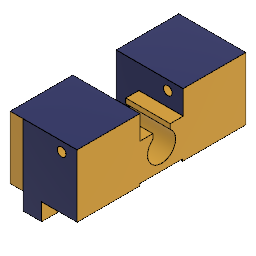
Lock_milling_jig_core_v1 v1 (Autodesk Fusion 360 design; units mm, degrees)
Autodesk Fusion 360 part; units mm, degrees
sketch "Sketch1" plane through (0, 0, 0) normal (0, 1, 0) x (1, 0, 0)
  line L0 (25, -14.9524) -> (-25, -14.9524)
  line L1 (-25, -14.9524) -> (-25, 0)
  line L2 (-25, 0) -> (25, 0)
  line L3 (25, 0) -> (25, -14.9524)
  constraint horizontal L0
  constraint vertical L1
  constraint horizontal L2
  constraint vertical L3
surface "Extrude1" add extruded along (0, 1, 0) between 0 and 50 path "Sketch1" along L2 L3 L0 L1 makes body 1
delete_face "SurfaceDeleteFace1" leaving the opening 1 faces at (8.3333, 16.6667, 14.9524) on bodies 1
delete_face "SurfaceDeleteFace2" leaving the opening 1 faces at (25, 16.6667, 4.9841) on bodies 1
delete_face "SurfaceDeleteFace3" leaving the opening 1 faces at (-8.3333, 16.6667, 0) on bodies 1
delete_face "SurfaceDeleteFace4" leaving the opening 1 faces at (-25, 16.6667, 9.9683) on bodies 1
sketch "Sketch2" plane through (0, 0, 0) normal (0, 1, 0) x (1, 0, 0)
  line L0 (-10, -10) -> (10, -10)
  line L1 (10, -10) -> (10, 0)
  line L2 (10, 0) -> (-10, 0)
  line L3 (-10, 0) -> (-10, -10)
  constraint horizontal L0
  constraint vertical L1
  constraint horizontal L2
  constraint vertical L3
extrude "Extrude2" add sketch "Sketch2" along normal mid plane 50 separate body makes body 2
hole "Hole1" at (-10, 0.0115, 9.2232) direction (1, 0, 0) diameter 12.9 depth 22 tip angle 180 bodies 2
hole "Hole2" at (0, 15.7073, 10) direction (0, 0, -1) diameter 4 depth 12 tip angle 118 counterbore diameter 6 counterbore depth 1 bodies 2
hole "Hole3" at (0, -15.6958, 10) direction (0, 0, -1) diameter 4 depth 12 tip angle 118 counterbore diameter 6 counterbore depth 1 bodies 2
sketch "Sketch3" plane through (0, 0, 0) normal (1, 0, 0) x (0, 1, 0)
  line L0 (6, 10, -10) -> (-6, 10, -10)
  line L1 (-6, 10, -10) -> (-6, 2, -10)
  line L2 (-6, 2, -10) -> (6, 2, -10)
  line L3 (6, 2, -10) -> (6, 10, -10)
extrude "Extrude3" cut sketch "Sketch3" along normal blind 10 contours L0 L1 L2 L3 in plane through (-10, 0, 0) normal (1, 0, 0) bodies 2
sketch "Sketch4" plane through (0, 0, 0) normal (0, 0, -1) x (1, 0, 0)
  circle A0 centre (0, 15.6958) radius 2
  circle A1 centre (0, -15.7073) radius 2
  line L0 (-10, 25) -> (-10, -25)
  line L1 (-10, -25) -> (10, -25)
  line L2 (10, -25) -> (10, 25)
  line L3 (10, 25) -> (-10, 25)
extrude "Extrude4" add 1 faces at (7.6639, 15.782, 10) along direction (0, 0, 1) blind 2 on bodies 2 bodies 2
extrude "Extrude5" add 1 faces at (7.6639, -15.6211, 10) along direction (0, 0, 1) blind 2 on bodies 2 bodies 2
extrude "Extrude6" cut 1 faces at (-6.6667, -2, 2) along direction (0, 0, -1) blind 1 on bodies 2 bodies 2
extrude "Extrude7" add sketch "Sketch4" along normal blind 2 bodies 2
chamfer "Chamfer1" distance 0.4 angle 45 1 edges at (-2.797, -14.6109, 12) on bodies 2
chamfer "Chamfer2" distance 0.4 angle 45 1 edges at (-2.797, 16.7921, 12) on bodies 2
chamfer "Chamfer3" distance 0.5 angle 45 1 edges at (-10, -25, 5) on bodies 2
chamfer "Chamfer4" distance 0.5 angle 45 1 edges at (10, -25, 5) on bodies 2
chamfer "Chamfer5" distance 0.5 angle 45 1 edges at (10, 25, 5) on bodies 2
chamfer "Chamfer6" distance 0.5 angle 45 1 edges at (-10, 25, 5) on bodies 2
sketch "Sketch5" plane through (0, 0, 0) normal (1, 0, 0) x (0, 1, 0)
  line L0 (10, 15) -> (-10, 15)
  line L1 (-10, 15) -> (-10, 1)
  line L2 (-10, 1) -> (10, 1)
  line L3 (10, 1) -> (10, 15)
  constraint horizontal L0
  constraint vertical L1
  constraint horizontal L2
  constraint vertical L3
extrude "Extrude8" cut sketch "Sketch5" against normal blind 12 bodies 2
extrude "Extrude9" add 1 faces at (7.2673, -4.9427, -2) along direction (0, 0, -1) blind 2 on bodies 2 bodies 2
chamfer "Chamfer7" distance 0.5 angle 45 1 edges at (-10, 10, 6.5) on bodies 2
chamfer "Chamfer8" distance 0.5 angle 45 1 edges at (-10, 0.25, 1) on bodies 2
chamfer "Chamfer9" distance 0.5 angle 45 1 edges at (-10, -10, 6.25) on bodies 2
extrude "Extrude10" add 1 faces at (3.3333, 6.4145, 10.6667) along direction (0, -1, 0) blind 2 on bodies 2 bodies 2
extrude "Extrude11" add 1 faces at (3.3333, -6.3916, 10.6667) along direction (0, 1, 0) blind 2 on bodies 2 bodies 2
extrude "Extrude12" add 1 faces at (7.7968, 14.7892, 12) along direction (0, 0, 1) blind 3 on bodies 2 bodies 2
extrude "Extrude13" add 1 faces at (7.7968, -14.7778, 12) along direction (0, 0, 1) blind 3 on bodies 2 bodies 2
sketch "Sketch6" plane through (10, 0, 0) normal (1, 0, 0) x (0, 1, 0)
  line L0 (24.5, -4) -> (24.5, 15)
  line L1 (24.5, 15) -> (4.4145, 15)
  line L2 (4.4145, 15) -> (4.4145, 10)
  line L3 (4.4145, 10) -> (6.4145, 10)
  arc A0 (-6.3916, 10) -> (6.4145, 10) centre (0.0115, 9.2232) ccw
  line L4 (-6.3916, 10) -> (-4.3916, 10)
  line L5 (-4.3916, 10) -> (-4.3916, 15)
  line L6 (-4.3916, 15) -> (-24.5, 15)
  line L7 (-24.5, 15) -> (-24.5, -4)
  line L8 (-24.5, -4) -> (24.5, -4)
  circle A1 centre (0.0115, 9.2232) radius 6.4
  constraint concentric A0 A1
extrude "Extrude14" cut sketch "Sketch6" against normal blind 19 contours L2 L3 A1 | L4 L5 A1 bodies 2
extrude "Extrude15" add 1 faces at (7.7968, 14.7892, 15) along direction (0, 0, 1) blind 4 on bodies 2 bodies 2
extrude "Extrude16" add 1 faces at (7.7968, -14.7778, 15) along direction (0, 0, 1) blind 4 on bodies 2 bodies 2
delete_face "DeleteFace1" 1 faces at (-9.6667, 10.1667, 10.6667) on bodies 2
delete_face "DeleteFace2" 1 faces at (-9.8333, -3.5, 0.6667) on bodies 2
delete_face "DeleteFace3" 1 faces at (-9.6667, -10.1667, 13) on bodies 2
delete_face "DeleteFace4" 1 faces at (-9.8333, 24.6667, 11.3333) on bodies 2
delete_face "DeleteFace5" 1 faces at (-9.8333, -24.6667, 3.6667) on bodies 2
extrude "Extrude17" add 1 faces at (-10, 20, 5.3333) along direction (-1, 0, 0) blind 8 on bodies 2 bodies 2
extrude "Extrude18" add 1 faces at (-13.1302, 16.9871, 19) along direction (0, 0, 1) blind 3 on bodies 2 bodies 2
extrude "Extrude19" add 1 faces at (-13.1302, -16.9833, 19) along direction (0, 0, 1) blind 3 on bodies 2 bodies 2
sketch "Sketch7" plane through (10, 0, 0) normal (1, 0, 0) x (0, 1, 0)
  arc A0 (6.3642, 10) -> (4.4145, 13.8679) centre (0.0115, 9.2232) ccw
  line L0 (-4.3916, 13.8679) -> (-4.3916, 22)
  line L1 (-4.3916, 22) -> (-24.5, 22)
  line L2 (-24.5, 22) -> (-24.5, -4)
  line L3 (-24.5, -4) -> (24.5, -4)
  line L4 (24.5, -4) -> (24.5, 22)
  line L5 (24.5, 22) -> (4.4145, 22)
  line L6 (4.4145, 22) -> (4.4145, 13.8679)
  line L7 (-8, 23) -> (8, 23)
  line L8 (8, 23) -> (8, 16)
  line L9 (8, 16) -> (-8, 16)
  line L10 (-8, 16) -> (-8, 23)
  line L11 (6.3642, 10) -> (6.4145, 10)
  arc A1 (-6.3916, 10) -> (6.4145, 10) centre (0.0115, 9.2232) ccw
  line L12 (-6.3916, 10) -> (-6.3412, 10)
  arc A2 (-4.3916, 13.8679) -> (-6.3412, 10) centre (0.0115, 9.2232) ccw
  constraint horizontal L7
  constraint vertical L8
  constraint horizontal L9
  constraint vertical L10
extrude "Extrude20" cut sketch "Sketch7" against normal blind 13 contours L5 L6 L8 L9 | L0 L1 L9 L10 bodies 2
hole "Hole4" at (-7.848, -25, 14.6725) direction (0, 1, 0) diameter 4 depth 50 tip angle 180 bodies 2
extrude "Extrude21" cut 1 faces at (-12.5508, -4.8564, -4) along direction (0, 0, 1) blind 2 on bodies 2 bodies 2
extrude "Extrude22" cut 1 faces at (-18, 20, 7) along direction (1, 0, 0) blind 3 on bodies 2 bodies 2
extrude "Extrude23" cut 1 faces at (6.6667, 8, 20) along direction (0, 1, 0) blind 2 on bodies 2 bodies 2
extrude "Extrude24" cut 1 faces at (6.6667, -8, 18) along direction (0, -1, 0) blind 2 on bodies 2 bodies 2
delete_face "DeleteFace6" 1 faces at (-7.6488, 15, 12.6824) on bodies 2
delete_face "DeleteFace7" 2 faces at (0, 13.7073, -1.3333) (2, 15.7073, 6) on bodies 2
delete_face "DeleteFace8" 2 faces at (0, -17.6958, -1.3333) (2, -15.6958, 6) on bodies 2
delete_face "DeleteFace9" 1 faces at (0.1695, -19.0916, 18.6667) on bodies 2
delete_face "DeleteFace10" 1 faces at (0.1695, 12.3115, 18.6667) on bodies 2
delete_face "DeleteFace11" 1 faces at (-7.6488, -20, 12.6824) on bodies 2
extrude "Extrude25" add 1 faces at (1.5, 15, 22) along direction (0, 0, 1) blind 4 on bodies 2 bodies 2
extrude "Extrude26" add 1 faces at (1.5, -15, 22) along direction (0, 0, 1) blind 5 on bodies 2 bodies 2
hole "Hole5" at (-9.451, -25, 21.8297) direction (0, 1, 0) diameter 4 depth 55 tip angle 118 bodies 2
extrude "Extrude27" add 1 faces at (0, -8.8121, 8.6844) along direction (-1, 0, 0) blind 9 on bodies 2 bodies 2
delete_face "DeleteFace12" 1 faces at (-10.9194, -20, 20.4719) on bodies 2
delete_face "DeleteFace13" 1 faces at (-10.9194, 20, 20.4719) on bodies 2
delete_face "DeleteFace14" 1 faces at (9.6667, -24.8333, 7.6667) on bodies 2
delete_face "DeleteFace15" 1 faces at (9.8333, 24.6667, 7.3333) on bodies 2
sketch "Sketch8" plane through (-15, 0, 0) normal (-1, 0, 0) x (0, -1, 0)
  line L0 (-25, -2) -> (25, -2)
  line L1 (25, -2) -> (25, 27)
  line L2 (25, 27) -> (10, 27)
  line L3 (10, 27) -> (10, 1)
  line L4 (10, 1) -> (-10, 1)
  line L5 (-10, 1) -> (-10, 26)
  line L6 (-10, 26) -> (-25, 26)
  line L7 (-25, 26) -> (-25, -2)
  line L8 (-25, -2) -> (25, -2)
  line L9 (25, -2) -> (25, -10)
  line L10 (25, -10) -> (-25, -10)
  line L11 (-25, -10) -> (-25, -2)
  constraint horizontal L8
  constraint vertical L9
  constraint horizontal L10
  constraint vertical L11
  constraint coincident L0.start L7.end
extrude "Extrude28" add sketch "Sketch8" against normal blind 9 contours L0 L8 L9 L10 L11 bodies 2
sketch "Sketch9" plane through (-15, 0, 0) normal (-1, 0, 0) x (0, -1, 0)
  line L0 (25, -10) -> (25, 27)
  line L1 (25, 27) -> (10, 27)
  line L2 (10, 27) -> (10, 1)
  line L3 (10, 1) -> (-10, 1)
  line L4 (-10, 1) -> (-10, 26)
  line L5 (-10, 26) -> (-25, 26)
  line L6 (-25, 26) -> (-25, -10)
  line L7 (-25, -10) -> (25, -10)
  line L8 (-10, -3) -> (10, -3)
  line L9 (10, -3) -> (10, -10)
  line L10 (10, -10) -> (-10, -10)
  line L11 (-10, -10) -> (-10, -3)
  constraint horizontal L8
  constraint vertical L9
  constraint horizontal L10
  constraint vertical L11
  constraint coincident L7 L9.end
extrude "Extrude29" cut sketch "Sketch9" against normal blind 17 contours L7 L8 L9 L10 L11 bodies 2
extrude "Extrude30" add 1 faces at (-9, -8.8121, 8.6844) along direction (-1, 0, 0) blind 1 on bodies 2 bodies 2
hole "Hole6" at (2.8828, -25, 22.6383) direction (0, 1, 0) diameter 4 depth 53 tip angle 118 bodies 2
extrude "Extrude31" cut 1 faces at (-12, 3.3333, -3) along direction (0, 0, 1) blind 1 on bodies 2 bodies 2
extrude "Extrude32" add 2 faces at (-9.5603, -25, 15.4638) (-12, -25, -4.6667) along direction (0, -1, 0) blind 14 on bodies 2 bodies 2
extrude "Extrude33" add 1 faces at (-6.5603, 25, 15.1304) along direction (0, 1, 0) blind 14 on bodies 2 bodies 2
extrude "Extrude34" cut 1 faces at (-12, 10, -4.6667) along direction (0, 1, 0) blind 13 on bodies 2 bodies 2
extrude "Extrude35" cut 1 faces at (-9, -10, -4.6667) along direction (0, -1, 0) blind 16 on bodies 2 bodies 2
extrude "Extrude36" cut 1 faces at (-10, -8.8121, 8.6844) along direction (1, 0, 0) blind 0.5 on bodies 2 bodies 2
hole "Hole7" at (-7.76, -6.4385, 9.2232) direction (0, -1, 0) diameter 8 depth 8 tip angle 118 bodies 2
sketch "Sketch10" plane through (10, 0, 0) normal (1, 0, 0) x (0, 1, 0)
  line L0 (39, 26) -> (10, 26)
  line L1 (10, 26) -> (10, 16)
  line L2 (10, 16) -> (4.4145, 16)
  line L3 (4.4145, 16) -> (4.4145, 13.8679)
  arc A0 (6.3642, 10) -> (4.4145, 13.8679) centre (0.0115, 9.2232) ccw
  line L4 (6.3642, 10) -> (6.4145, 10)
  arc A1 (-6.3916, 10) -> (6.4145, 10) centre (0.0115, 9.2232) ccw
  line L5 (-6.3916, 10) -> (-6.3412, 10)
  arc A2 (-4.3916, 13.8679) -> (-6.3412, 10) centre (0.0115, 9.2232) ccw
  line L6 (-4.3916, 13.8679) -> (-4.3916, 16)
  line L7 (-4.3916, 16) -> (-10, 16)
  line L8 (-10, 16) -> (-10, 27)
  line L9 (-10, 27) -> (-39, 27)
  line L10 (-39, 27) -> (-39, -2)
  line L11 (-39, -2) -> (39, -2)
  line L12 (39, -2) -> (39, 26)
  line L13 (-10, 16) -> (10, 16)
  line L14 (10, 16) -> (10, 1)
  line L15 (10, 1) -> (-10, 1)
  line L16 (-10, 1) -> (-10, 16)
  constraint horizontal L13
  constraint vertical L14
  constraint horizontal L15
  constraint vertical L16
  constraint coincident L7.end L8.start
extrude "Extrude37" cut sketch "Sketch10" against normal blind 26 contours L2 L3 A0 L4 A1 L5 A2 L6 L7 L13 L14 L15 L16 | L3 A0 L4 A1 L5 A2 L6 L13 bodies 2
delete_face "DeleteFace16" 1 faces at (-11.76, -12.959, 9.2232) on bodies 2
sketch "Sketch11" plane through (10, 0, 0) normal (1, 0, 0) x (0, 1, 0)
  line L0 (10, 26) -> (10, 1)
  line L1 (10, 1) -> (-10, 1)
  line L2 (-10, 1) -> (-10, 27)
  line L3 (-10, 27) -> (-39, 27)
  line L4 (-39, 27) -> (-39, -2)
  line L5 (-39, -2) -> (39, -2)
  line L6 (39, -2) -> (39, 26)
  line L7 (39, 26) -> (10, 26)
  line L8 (-10, 15.9908) -> (10, 15.9908)
  line L9 (10, 15.9908) -> (10, 1)
  line L10 (10, 1) -> (-10, 1)
  line L11 (-10, 1) -> (-10, 15.9908)
  constraint horizontal L8
  constraint vertical L9
  constraint horizontal L10
  constraint vertical L11
  constraint coincident L0.end L1.start
  constraint coincident L2 L8.start
extrude "Extrude38" add sketch "Sketch11" against normal blind 20.5 contours L0 L1 L2 L8 L9 L10 L11 bodies 2
sketch "Sketch12" plane through (10, 0, 0) normal (1, 0, 0) x (0, 1, 0)
  line L0 (10, 26) -> (10, 15.9908)
  line L1 (10, 15.9908) -> (-10, 15.9908)
  line L2 (-10, 15.9908) -> (-10, 27)
  line L3 (-10, 27) -> (-39, 27)
  line L4 (-39, 27) -> (-39, -2)
  line L5 (-39, -2) -> (39, -2)
  line L6 (39, -2) -> (39, 26)
  line L7 (39, 26) -> (10, 26)
  line L8 (-4, 20) -> (4, 20)
  line L9 (4, 20) -> (4, 12)
  line L10 (4, 12) -> (-4, 12)
  line L11 (-4, 12) -> (-4, 20)
  constraint horizontal L8
  constraint vertical L9
  constraint horizontal L10
  constraint vertical L11
extrude "Extrude39" cut sketch "Sketch12" against normal blind 27 contours L1 L9 L10 L11 bodies 2
hole "Hole8" at (10, 0.0064, 8.5976) direction (-1, 0, 0) diameter 12.95 depth 25 tip angle 118 bodies 2
extrude "Extrude40" cut 1 faces at (-6, 33.6667, -4.6667) along direction (-1, 0, 0) blind 0.4 on bodies 2 bodies 2
extrude "Extrude41" cut 1 faces at (-6, -34.6667, -7.3333) along direction (-1, 0, 0) blind 0.4 on bodies 2 bodies 2
extrude "Extrude42" cut 1 faces at (-12.1333, 23, -7.3333) along direction (0, 1, 0) blind 2 on bodies 2 bodies 2
extrude "Extrude43" add 1 faces at (-12.1333, -26, -4.6667) along direction (0, 1, 0) blind 1 on bodies 2 bodies 2
extrude "Extrude44" add 1 faces at (1.6667, 19.6667, 26) along direction (0, 0, 1) blind 1 on bodies 2 bodies 2
sketch "Sketch13" plane through (-15, 0, 0) normal (-1, 0, 0) x (0, -1, 0)
  line L0 (-25, -2) -> (25, -2)
  line L1 (25, -2) -> (25, -10)
  line L2 (25, -10) -> (39, -10)
  line L3 (39, -10) -> (39, 27)
  line L4 (39, 27) -> (10, 27)
  line L5 (10, 27) -> (10, 1)
  line L6 (10, 1) -> (-10, 1)
  line L7 (-10, 1) -> (-10, 27)
  line L8 (-10, 27) -> (-39, 27)
  line L9 (-39, 27) -> (-39, -10)
  line L10 (-39, -10) -> (-25, -10)
  line L11 (-25, -10) -> (-25, -2)
  line L12 (-25, -2) -> (-39, -2)
  line L13 (-39, -2) -> (-39, -10)
  line L14 (-39, -10) -> (-25, -10)
  line L15 (-25, -10) -> (-25, -2)
  line L16 (25, -2) -> (39, -2)
  line L17 (39, -2) -> (39, -10)
  line L18 (39, -10) -> (25, -10)
  line L19 (25, -10) -> (25, -2)
  constraint horizontal L12
  constraint vertical L13
  constraint horizontal L14
  constraint vertical L15
  constraint coincident L9.end L10.start
  constraint coincident L0.start L11.end
  constraint horizontal L16
  constraint vertical L17
  constraint horizontal L18
  constraint vertical L19
  constraint coincident L2.end L3.start
  constraint coincident L0.end L1.start
extrude "Extrude45" add sketch "Sketch13" along normal blind 6 contours L0 L3 L4 L5 L6 L7 L8 L9 L12 L16 bodies 2
sketch "Sketch14" plane through (0, 0, -2) normal (0, 0, -1) x (1, 0, 0)
  line L0 (-6.4, 25) -> (-15, 25)
  line L1 (-15, 25) -> (-15, 39)
  line L2 (-15, 39) -> (-21, 39)
  line L3 (-21, 39) -> (-21, -39)
  line L4 (-21, -39) -> (-15, -39)
  line L5 (-15, -39) -> (-15, -25)
  line L6 (-15, -25) -> (-6.4, -25)
  line L7 (-6.4, -25) -> (-6.4, -39)
  line L8 (-6.4, -39) -> (10, -39)
  line L9 (10, -39) -> (10, 39)
  line L10 (10, 39) -> (-6.4, 39)
  line L11 (-6.4, 39) -> (-6.4, 25)
  line L12 (-21, -9.7105) -> (10, -9.7105)
  line L13 (10, -9.7105) -> (10, 10)
  line L14 (10, 10) -> (-21, 10)
  line L15 (-21, 10) -> (-21, -9.7105)
  constraint horizontal L12
  constraint vertical L13
  constraint horizontal L14
  constraint vertical L15
  constraint coincident L9 L13.end
  constraint coincident L3 L12.start
extrude "Extrude46" cut sketch "Sketch14" against normal blind 1 contours L3 L9 L12 L13 L14 L15 bodies 2
form "Form1" [no effect]
